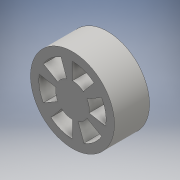
# Autodesk Inventor part: Small Flywheel
Saved by Autodesk Inventor 2016 (Build 200138000, 138)
## iProperties
Created: 2015-12-24
Part Number: Small Flywheel
Material: Generic
Document SubType Name: Modeling
Designer: jonathan
Density: 1 g/cm^3
Appearance: Default
Author: jonathan
Autodesk Inventor part; units mm, degrees
ref_plane "YZ Plane" through (0, 0, 0) normal (1, 0, 0) x (0, 1, 0)
ref_plane "XZ Plane" through (0, 0, 0) normal (0, 1, 0) x (-1, 0, 0)
ref_plane "XY Plane" through (0, 0, 0) normal (0, 0, 1) x (1, 0, 0)
sketch "Sketch1" plane through (0, 0, 0) normal (0, 1, 0) x (-1, 0, 0)
  circle A0 centre (0, 0) radius 30
  dimension "d0" = 60
  constraints: 1 centre point, 1 coincident
  measures "d0" diameter of A0
extrude "Extrusion1" add sketch "Sketch1" along normal blind 25
sketch "Sketch2" plane through (0, 0, 0) normal (0, -1, 0) x (1, 0, 0)
  line L0 (0, 0) -> (0, 24)
  arc A0 (15.4269, 18.3851) -> (0, 24) centre (0, 0) ccw
  arc A1 (7.7135, 9.1925) -> (0, 12) centre (0, 0) ccw
  line L1 (0, 0) -> (15.4269, 18.3851)
  dimension "d3" = 40
  dimension "d4" = 12
  dimension "d5" = 24
  constraints: 4 end point, 4 point on circle, 2 centre point, 2 coincident, 2 midpoint, 1 vertical
  measures "d3" angle of L0 L1
  measures "d4" radius of A1
  measures "d5" radius of A0
extrude "Extrusion2" cut sketch "Sketch2" against normal through all contours L0 A0 L1 A1
pattern_circular "Circular Pattern1" count 6 over 360 about axis through (0, 0, 0) along (0, 1, 0) of "Extrusion2"
body "Solid1"
